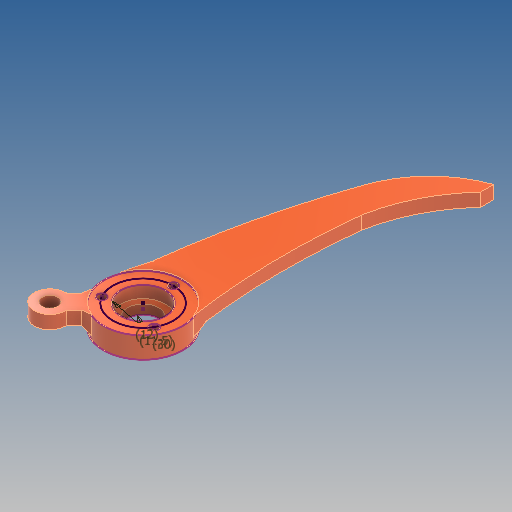
# Autodesk Inventor part: 01-03-01 Zange links nue
Saved by Autodesk Inventor 2026.2 (Build 302298000, 298)
## iProperties
Created: 2025-12-11
Part Number: 01-03-01 Zange links nue
Material: Phenolharz
Document SubType Name: Modeling
Designer: Schally
Density: 1.38 g/cm^3
Appearance: Glatt - Hellorange
Author: Schally
Autodesk Inventor part; units mm, degrees
sketch "Skizze10" plane through (0, 0, 0) normal (1, 0, 0) x (0, 1, 0)
  line L0 (-1.4, 0) -> (8.4, 0) projected
  line L1 (0, -13.2) -> (0, 2.2) projected
  line L2 (2, -2.5) -> (7, -2.5)
  line L3 (7, -2.5) -> (7, -8)
  line L4 (7, -8) -> (2, -8)
  line L5 (2, -8) -> (2, -2.5)
  point P0 (0, 0)
  point P1 (0, -11)
  dimension "d135" = 8
  dimension "d137" = 5
  dimension "d138" = 2
  dimension "d145" = 2.5
  constraints: 8 end point, 2 parallel, 1 horizontal, 1 perpendicular, 1 point on line
  measures "d135" distance between parallel lines of L0 L4
  measures "d137" distance between parallel lines of L5 L3
  measures "d138" distance between parallel lines of L1 L5
  measures "d145" distance between parallel lines of L0 L2
revolve "Umdrehung2" add sketch "Skizze10" angle 360 about axis through (0, -10, 0) along (0, 1, 0)
ref_plane "Arbeitsebene2" through (0, 6, 0) normal (0, 1, 0) x (1, 0, 0)
ref_plane "Arbeitsebene3" through (0, 4.5, 0) normal (0, 1, 0) x (1, 0, 0)
sketch "Skizze12" plane through (0, 4.5, 0) normal (0, 1, 0) x (1, 0, 0)
  arc A0 (3.5, 80) -> (-11.5, 15.25) centre (296.2619, -21.9337) ccw projected
  arc A1 (28, 100) -> (13, 70) centre (72.0267, 59.2367) ccw projected
  line L0 (28, 100) -> (28, 105) projected
  arc A2 (28, 105) -> (3.5, 80) centre (41.4387, 67.3251) ccw projected
  circle A3 centre (0, 0) radius 15
  arc A4 (13, 70) -> (15, 0) centre (261.1443, 42.0613) ccw
  arc A5 (-11.5, 15.25) -> (-15, 0) centre (120.624, -23.1002) ccw
  circle A6 centre (0, 0) radius 8 projected
  line L1 (0, 0) -> (-17.6777, -17.6777)
  line L2 (-78.9324, 0) -> (358.7942, 0) projected
  line L3 (0, 133.8507) -> (0, -48.3491) projected
  circle A7 centre (-17.6777, -17.6777) radius 6
  circle A8 centre (-17.6777, -17.6777) radius 3
  line L4 (2.8284, -2.8284) -> (-11.687, -17.3438)
  line L5 (-2.8284, 2.8284) -> (-17.3438, -11.687)
  point P0 (-16.4, 0)
  point P1 (-13.051, -7.3941)
  point P2 (-10.4814, -11.4821)
  point P3 (-7.2048, -13.7764)
  point P4 (-7.3941, -13.051)
  point P5 (14.2414, 4.7098)
  dimension "d147" = 30
  dimension "d148" = 45
  dimension "d149" = 25
  dimension "d150" = 12
  dimension "d152" = 3
  dimension "d153" = 4
  dimension "d154" = 4
  constraints: 8 point on circle, 6 end point, 5 centre point, 3 coincident, 2 parallel
  measures "d147" diameter of A3
  measures "d148" angle of L1 L3
  measures "d149" distance of L1.start L1.end
  measures "d150" diameter of A7
  measures "d152" radial gap between concentric circles of A7 A8
  measures "d153" distance between parallel lines of L1 L4
  measures "d154" distance between parallel lines of L1 L5
sketch "Skizze13" plane through (0, 4.5, 0) normal (0, 1, 0) x (1, 0, 0)
  point P0 (0, 0)
extrude "Extrusion8" add sketch "Skizze12" along normal mid plane 5 contours A2 L0 A1 A4 A3 L3 A0 | L3 A3 A5 A0 | L3 A6 L2 A5 A3 | A3 A4 L2 A6 L3 | A3 A4 | L3 L2 A6 | A6 L2 L3 | L2 A6 L5 A3 | A3 L3 A6 L2 | A6 L3 L2 | L2 L5 A6 | L3 L4 A6 L1 | L1 A6 L5 L2 | L5 A6 L1 A3 | A3 L1 A7 L5 | A3 L4 A6 L3 | A6 L4 L3 | A6 L4 A3 L1 | A3 L4 A7 L1 | A7
sketch "Skizze15" plane through (0, 4.5, 0) normal (0, 1, 0) x (1, 0, 0)
  arc A0 (-11.5, 15.25) -> (-15, 0) centre (120.624, -23.1002) ccw projected
  circle A1 centre (0, 0) radius 15
  constraints: 1 coincident, 1 horizontal alignment, 2 other
extrude "Extrusion10" add sketch "Skizze15" along normal mid plane 12
sketch "Skizze16" plane through (0, 4.5, 0) normal (0, 1, 0) x (1, 0, 0)
  circle A0 centre (0, 0) radius 6
  dimension "d162" = 12
  constraints: 1 centre point, 1 coincident
  measures "d162" diameter of A0
extrude "Extrusion11" cut sketch "Skizze16" along normal mid plane 12
sketch "Skizze17" plane through (0, 4.5, 0) normal (0, 1, 0) x (1, 0, 0)
  circle A0 centre (0, 0) radius 8.5
  dimension "d165" = 17
  constraints: 1 centre point, 1 coincident
  measures "d165" diameter of A0
extrude "Extrusion12" cut sketch "Skizze17" along normal mid plane 5
chamfer "Fasen7" distance 2 angle 45 8 edges at (-10.6066, 7, 10.6066) (-7.3941, 5.75, 13.051) (-7.3941, 3.25, 13.051) (-10.6066, 2, 10.6066) (0.4428, 2, -14.9935) (0.4428, 7, -14.9935) (-13.051, 5.75, 7.3941) (-13.051, 3.25, 7.3941)
ref_plane "Arbeitsebene4" through (0, 4.5, 0) normal (0, 1, 0) x (1, 0, 0)
sketch "Skizze21" plane through (0, 10.5, 0) normal (0, 1, 0) x (1, 0, 0)
  circle A0 centre (0, 0) radius 15
  dimension "d200" = 30
  constraints: 1 centre point, 1 coincident
  measures "d200" diameter of A0
extrude "Extrusion16" cut sketch "Skizze21" against normal blind 4
sketch "Skizze23" plane through (0, 6.5, 0) normal (0, 1, 0) x (1, 0, 0)
  line L0 (-34.0132, 0) -> (38.3355, 0) projected
  line L1 (0, 130.7355) -> (0, -49.4132) projected
  line L2 (0, 0) -> (0, 20.1991)
  line L3 (0, 0) -> (-17.4929, -10.0995)
  line L4 (0, 0) -> (17.4929, -10.0995)
  circle A0 centre (0, 0) radius 8.5 projected
  arc A1 (14.2414, 4.7098) -> (-13.9387, 5.5419) centre (0, 0) ccw projected
  circle A2 centre (0, 0) radius 11.5
  circle A3 centre (-9.9593, -5.75) radius 1.6
  circle A4 centre (9.9593, -5.75) radius 1.6
  circle A5 centre (0, 11.5) radius 1.6
  arc A6 (-5.5921, -13.9186) -> (14.2414, 4.7098) centre (0, 0) ccw projected
  arc A7 (-13.9387, 5.5419) -> (-13.9186, -5.5921) centre (0, 0) ccw projected
  arc A8 (-13.9186, -5.5921) -> (-5.5921, -13.9186) centre (0, 0) ccw projected
  dimension "d203" = 360
  dimension "d205" = 3
  dimension "d206" = 3.2
  dimension "d207" = 3.2
  dimension "d208" = 3.2
  constraints: 6 end point, 4 centre point, 4 point on line, 3 point on circle, 2 coincident, 8 other
  measures "d205" radial gap between concentric circles of A0 A2
  measures "d206" diameter of A3
  measures "d207" diameter of A4
  measures "d208" diameter of A5
extrude "Extrusion17" cut sketch "Skizze23" against normal blind 8 contours A5 A2 L1 | L1 A2 A5 | A3 A2 L3 | L3 A2 A3 | A4 A2 L4 | L4 A2 A4 | A2 L1 A5 | A4 L4 A2 | A5 L1 A2 | A2 L3 A3 | A3 L3 A2 | A2 L4 A4
sketch "Skizze24" plane through (0, -1.5, 0) normal (0, -1, 0) x (1, 0, 0)
  circle A0 centre (0, -11.5) radius 1.6 projected
  circle A1 centre (9.9593, 5.75) radius 1.6 projected
  circle A2 centre (-9.9593, 5.75) radius 1.6 projected
  circle A3 centre (0, 0) radius 6 projected
  circle A4 centre (0, 0) radius 15 projected
  dimension "d211" = 12
  dimension "d212" = 30
  dimension "d213" = 11.5
  measures "d211" diameter of A3
  measures "d212" diameter of A4
  measures "d213" distance of point (0, 0) A1.centre
sketch "Skizze25" plane through (28, 7, -100) normal (0, 1, 0) x (1, 0, 0)
  line L0 (-56.3412, -125.0488) -> (1.0248, -125.0488)
  line L1 (1.0248, -125.0488) -> (1.0248, -72.2498)
  line L2 (1.0248, -72.2498) -> (-56.3412, -72.2498)
  line L3 (-56.3412, -72.2498) -> (-56.3412, -125.0488)
  constraints: 8 end point, 2 parallel, 1 horizontal, 1 perpendicular
extrude "Extrusion18" cut sketch "Skizze25" along normal blind 10
sketch "Skizze26" plane through (0, 6.5, 0) normal (0, 1, 0) x (1, 0, 0)
  circle A0 centre (0, 11.5) radius 1.6 projected
  circle A1 centre (9.9593, -5.75) radius 1.6 projected
  circle A2 centre (-9.9593, -5.75) radius 1.6 projected
  circle A3 centre (0, 0) radius 8.5 projected
  arc A4 (-5.5921, -13.9186) -> (14.2414, 4.7098) centre (0, 0) ccw projected
  arc A5 (14.2414, 4.7098) -> (-13.9387, 5.5419) centre (0, 0) ccw projected
  arc A6 (-13.9387, 5.5419) -> (-13.9186, -5.5921) centre (0, 0) ccw projected
  arc A7 (-13.9186, -5.5921) -> (-5.5921, -13.9186) centre (0, 0) ccw projected
  circle A8 centre (0, 0) radius 11.5
  constraints: 1 coincident, 1 vertical alignment, 2 other
sketch "Skizze27" plane through (0, -1.5, 0) normal (0, -1, 0) x (1, 0, 0)
  circle A0 centre (0, -11.5) radius 1.6 projected
  circle A1 centre (9.9593, 5.75) radius 1.6 projected
  circle A2 centre (-9.9593, 5.75) radius 1.6 projected
  circle A3 centre (9.9593, 5.75) radius 2.1
  circle A4 centre (-9.9593, 5.75) radius 2.1
  circle A5 centre (0, -11.5) radius 2.1
  dimension "d216" = 4.2
  dimension "d217" = 4.2
  dimension "d218" = 4.2
  constraints: 3 centre point, 3 coincident
  measures "d216" diameter of A3
  measures "d217" diameter of A4
  measures "d218" diameter of A5
extrude "Extrusion19" cut sketch "Skizze27" against normal blind 6 contours A0 | A1 | A2 | A3 | A4 | A5
